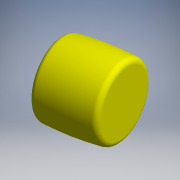
# Autodesk Inventor part: 21308 E_r2
Saved by Autodesk Inventor 2017.3 (Build 213256000, 256)
## iProperties
Part Number: 21308 E_r2
Material: Generic
Catalog Web Link: www.cadenas.de
Description: BS2_001-Spherical roller bearings
Vendor: SKF
Document SubType Name: Modeling
Designer: partserver
Manufacturer: SKF
Mass: 0.661349 g
Surface Area: 3.9938 cm^2
Volume: 0.661349 cm^3
Density: 1 g/cm^3
Appearance: PSOLRGB-255-255-0
Category: PARTsolutions
Company: SKF
Title: 21308 E_r2
Author: Cadenas PARTsolutions
Comments: Spherical roller bearings
PSOL_IDENT_0: {$CADENAS_DATA\23d-libs\skf\bearings_units_and_housings\roller_bearings\spherical_roller_bearings\pa
PSOL_IDENT_1: rts\bs2_001_roller2.prj},165 {VTYP=3D},{NB=21308 E_r2},{LINA=21308 E_r2},{NN=BS2_001},{DATE=23.12.20
PSOL_IDENT_2: 20 11:58:31},{GEOMDATE=24.11.2020 12:16:09},{VERSION=},{LINEID=461840},{WBVAR=},{WBNUMERIC=}  {NB=21
PSOL_IDENT_3: 308 E_r2},{LINA=21308 E_r2},{KT=DUMMY},{DESIGNATION=21308 E},{VARIANT=CE1W33},{DESIGNX=Cylindrical b
PSOL_IDENT_4: ore},{SEAL=No seals},{SALG=NO},{BORE=40.000},{DD=40.000},{DD1=MIN},{D=90.000},{B=23.000},{DD2=60.000
PSOL_IDENT_5: },{DD3=MIN},{D1=79.800},{B1=MIN},{B2=MIN},{B4=MIN},{B5=MIN},{BB=5.500},{K=3.000},{R12=1.500},{G=},{G
PSOL_IDENT_6: 1=MIN},{TB=MIN},{ALPHA=9.0833},{R34=MIN},{PITCH=71.097},{DW=10.200},{LW=8.400},{DDAMIN=49.000},{DDAM
PSOL_IDENT_7: AX=MIN},{DBMIN=MIN},{DAMAX=81.000},{BAMIN=MIN},{RAMAX=1.500},{LOAD1=107.000},{LOAD2=108.000},{LOAD3=
PSOL_IDENT_8: 11.800},{SPEED1=7000},{SPEED2=9500},{PRA=},{PLA=},{Z=19.000},{II=2.000},{MASS=0.740},{MASS2=MIN},{SL
PSOL_IDENT_9: EEVE=},{POPULAR=Yes},{BEARING=21308 E},{PPATH=parts/bs2_001_asmtpl.prj},{RAMAXX=1.5},{EE=0.24},{Y0=2
PSOL_IDENT_10: .8},{R12X=1.5},{Y2=4.2},{ALPHAX=9.08333},{Y1=2.8},{DD1X=},{B1X=},{SLEEVEX=},{ALPHAXX=},{B2X=},{SUPRE
PSOL_IDENT_11: SSED=},{BBALG=5.500},{KALG=3.000}
NB: 21308 E_r2
NN: BS2_001
NT: Spherical roller bearings
NBSYN: $DESIGNATION._r2
LINA: 21308 E_r2
CATALOG: SKF
DESIGNATION: 21308 E
VARIANT: CE1W33
DESIGNX: Cylindrical bore
SEAL: No seals
BORE: 40
DD: 40
DD1: 0
D: 90
B: 23
DD2: 60
DD3: 0
D1: 79.8
B1: 0
B2: 0
B4: 0
B5: 0
BB: 5.5
K: 3
R12: 1.5
G1: 0
TB: 0
ALPHA: 9.0833
R34: 0
PITCH: 71.097
DW: 10.2
LW: 8.4
DDAMIN: 49
DDAMAX: 0
DBMIN: 0
DAMAX: 81
BAMIN: 0
RAMAX: 1.5
LOAD1: 107
LOAD2: 108
LOAD3: 11.8
SPEED1: 7000
SPEED2: 9500
Z: 19
II: 2
MASS: 0.74
MASS2: 0
POPULAR: Yes
BEARING: 21308 E
PPATH: parts/bs2_001_asmtpl.prj
RAMAXX: 1.5
EE: 0.24
Y0: 2.8
R12X: 1.5
Y2: 4.2
ALPHAX: 9.08333
Y1: 2.8
SUPPLIER: SKF
ARTICLENO: 21308 E_r2
BOMINFO: 21308 E_r2
CREATOR: CADENAS GmbH
Autodesk Inventor part; units mm, degrees
sketch "Sketch_1" plane through (0, 0, 0) normal (0, 0, 1) x (1, 0, 0)
  line L0 (21.3728, 34.7471) -> (13.1272, 36.3499)
  line L1 (13.1272, 36.3499) -> (13.9287, 40.4733)
  arc A0 (14.7438, 41.076) -> (13.9287, 40.4733) centre (14.6649, 40.3302) ccw
  arc A1 (21.6443, 39.7347) -> (14.7438, 41.076) centre (10.467, 0.6531) ccw
  arc A2 (22.1743, 38.8705) -> (21.6443, 39.7347) centre (21.4381, 39.0136) ccw
  line L2 (22.1743, 38.8705) -> (21.3728, 34.7471)
  line L3 (21.3728, 34.7471) -> (13.1272, 36.3499)
  constraints: 8 end point, 6 point on circle, 3 centre point
revolve "Revolution1" add sketch "Sketch_1" angle 360 about axis through (21.3728, 34.7471, 0) along (0.9816272, -0.190809, 0)
ref_plane "NO_GEO_XY" through (0, 0, 0) normal (1, 0, 0) x (0, 0, -1)
ref_plane "NO_GEO_YZ" through (0, 0, 0) normal (0, 0, -1) x (0, 1, 0)
ref_plane "NO_GEO_ZX" through (0, 0, 0) normal (0, 1, 0) x (1, 0, 0)
ref_plane "roller2_XY" through (0, 35.5485, 0) normal (1, 0, 0) x (0, 0, -1)
ref_plane "roller2_YZ" through (0, 35.5485, 0) normal (0, 0, -1) x (0, 1, 0)
ref_plane "roller2_ZX" through (0, 35.5485, 0) normal (0, 1, 0) x (1, 0, 0)
body "Solid1"
